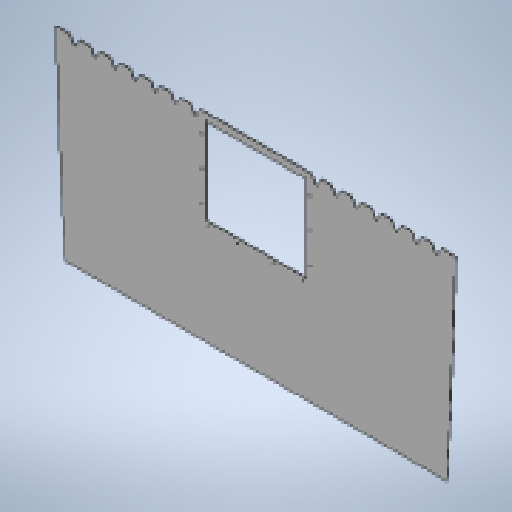
# Autodesk Inventor part: MSC 705 ridge 3
Saved by Autodesk Inventor 2025 (Build 290162010, 162A)
## iProperties
Created: 2024-06-08
Part Number: MSC 705 ridge 3
Material: Stainless Steel
Document SubType Name: Sheet Metal
Designer: admin
Density: 8 g/cm^3
Sheet Metal Rule: AISI304 2mm Die16
Appearance: Default
Stock Number: МОО 705 гребень 3
Flat Pattern Width: 79 cm
Flat Pattern Length: 159 cm
Flat Pattern Area: 12561 cm^2
Sheet Metal Width: 790,000 mm
Sheet Metal Length: 1590,000 mm
Sheet Metal Area: 1256100,000 mm^2
Author: admin
Autodesk Inventor part; units mm, degrees
ref_plane "YZ Plane" through (0, 0, 0) normal (1, 0, 0) x (0, 1, 0)
ref_plane "XZ Plane" through (0, 0, 0) normal (0, 1, 0) x (-1, 0, 0)
ref_plane "XY Plane" through (0, 0, 0) normal (0, 0, 1) x (1, 0, 0)
sketch "Sketch1" plane through (0, 0, 0) normal (0, 1, 0) x (-1, 0, 0)
  line L0 (-900, 0) -> (-900, -513)
  line L1 (-900, -513) -> (-830.3307, -790)
  line L2 (0, -790) -> (0, 0)
  line L3 (0, 0) -> (-900, 0)
  line L4 (0, -370) -> (-200, -370)
  line L5 (-200, -370) -> (-200, 0)
  line L6 (-830.3307, -790) -> (0, -790)
  line L7 (-200, -30) -> (0, -30)
  arc A0 (-795, 0) -> (-760, -790) centre (19673.6209, 511.0623) ccw
  dimension "d0" = 513
  dimension "d2" = 790
  dimension "d6" = 200
  dimension "d19" = 370
  dimension "d23" = 900
  dimension "d43" = 30
  dimension "d58" = 760
  dimension "d59" = 790
  dimension "d60" = 795
  dimension "d61" = 20475
  measures "d0" distance of L0.start L0.end
  measures "d2" distance of L2.start L2.end
  measures "d6" distance between parallel lines of L2 L5
  measures "d19" distance of L4.end L5.end
  measures "d23" distance between parallel lines of L0 L2
  measures "d43" distance between parallel lines of L7 L3
  measures "d58" distance of L2.start A0.end
  measures "d59" distance between parallel lines of L3 L6
  measures "d60" distance of L2.end A0.start
  measures "d61" radius of A0
extrude "Plate1" add sketch "Sketch1" along normal blind 2 contours L3 L5 L4 L2 L6 A0 | L3 L2 L7 L5
sketch "Sketch5" plane through (0, 2, 0) normal (0, 1, 0) x (1, 0, 0)
  line L0 (795, 0) -> (0, 0) projected
  line L1 (0, 790) -> (760, 790) projected
  line L2 (0, 370) -> (0, 790) projected
  line L3 (200, 370) -> (0, 370) projected
  line L4 (200, 30) -> (200, 370) projected
  line L5 (0, 0) -> (795, 0) projected
  line L6 (220, 0) -> (237.5, 30)
  line L7 (237.5, 30) -> (242.5, 30)
  line L8 (242.5, 30) -> (260, 0)
  line L9 (0, 30) -> (200, 30) projected
  line L10 (0, 0) -> (0, 30) projected
  arc A0 (795, 0) -> (760, 790) centre (-19673.6209, -511.0623) ccw projected
  point P0 (900, 0)
  point P1 (260, 0)
  dimension "d34" = 30
  dimension "d35" = 5
  dimension "d36" = 40
  dimension "d44" = 20
  constraints: 6 end point, 2 point on line, 1 equal length, 1 parallel
  measures "d34" distance between parallel lines of L7 L0
  measures "d35" distance of L6.end L7.end
  measures "d36" distance of L6.start L8.end
  measures "d44" distance from line of L6.start L4
extrude "Extrusion1" cut sketch "Sketch5" against normal through all contours L0 L6 L7 L8
pattern_linear "Rectangular Pattern1" count 7 spacing 80 along (1, 0, 0) of "Extrusion1"
sketch "Sketch7" plane through (0, 2, 0) normal (0, 1, 0) x (1, 0, 0)
  line L0 (215, 80) -> (215, 320) construction
  line L1 (190, 385) -> (70, 385) construction
  line L2 (200, 30) -> (200, 370) construction
  line L3 (200, 370) -> (0, 370) construction
  line L4 (0, 790) -> (0, 370) projected
  point P0 (0, 0)
  point P1 (215, 200)
  point P2 (200, 200)
  dimension "d45" = 15
  dimension "d46" = 240
  dimension "d47" = 10
  dimension "d48" = 15
  dimension "d49" = 190
  dimension "d50" = 120
  dimension "d62" = 70
  constraints: 4 coincident, 4 end point, 2 midpoint, 1 horizontal, 1 horizontal alignment, 1 vertical
  measures "d45" distance between parallel lines of L0 L2
  measures "d46" distance of L0.start L0.end
  measures "d47" distance from line of point (190, 385) L2
  measures "d48" distance between parallel lines of L1 L3
  measures "d49" horizontal distance of L3.end point (190, 385)
  measures "d50" distance of point (190, 385) point (70, 385)
  measures "d62" distance from line of point (70, 385) L4
hole "Hole1" at (215, 2, -80) at (215, 2, -200) at (215, 2, -320) at (190, 2, -385) at (70, 2, -385) direction (0, -1, 0) diameter 5.1 end through all
mirror "Mirror1" about plane through (0, 0, 0) normal (1, 0, 0) of "Plate1", "Extrusion1", "Rectangular Pattern1", "Hole1"
equation "\"d48\" = d45"
equation "\"d56\" = Thickness"
equation "\"d3\" = Thickness"
equation "\"BendReliefWidth\" = Thickness"
equation "\"BendReliefDepth\" = 0.5 * Thickness"
equation "\"CornerReliefSize\" = 4 * Thickness"
equation "\"MinimumRemnant\" = 2 * Thickness"
equation "\"GapSize\" = Thickness"
equation "\"Thickness\" = 2"
body "Solid1"
